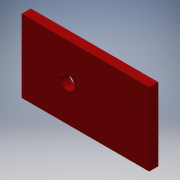
# Autodesk Inventor part: Gripper Piston
Saved by Autodesk Inventor 2016 (Build 200138000, 138)
## iProperties
Created: 2015-06-19
Part Number: Gripper Piston
Material: Aluminum 6061
Document SubType Name: Modeling
Designer: steele
Density: 2.7 g/cm^3
Appearance: Red
Mass: 71.2341 g
Surface Area: 102.839 cm^2
Volume: 26.383 cm^3
Author: steele
Autodesk Inventor part; units mm, degrees
ref_plane "YZ Plane" through (0, 0, 0) normal (1, 0, 0) x (0, 1, 0)
ref_plane "XZ Plane" through (0, 0, 0) normal (0, 1, 0) x (-1, 0, 0)
ref_plane "XY Plane" through (0, 0, 0) normal (0, 0, 1) x (1, 0, 0)
sketch "Sketch2" plane through (0, 0, 0) normal (0, 0, 1) x (1, 0, 0)
  line L0 (0, 0) -> (-31.75, 0) construction
  line L1 (-31.75, 0) -> (-31.75, -25.4)
  line L2 (-31.75, 0) -> (-31.75, 25.4)
  line L3 (-31.75, 25.4) -> (57.15, 25.4)
  line L4 (0, 0) -> (0, -25.4) construction
  line L5 (0, 0) -> (57.15, 0) construction
  line L6 (-31.75, -25.4) -> (57.15, -25.4)
  line L7 (57.15, 25.4) -> (57.15, -25.4)
  dimension "edgeToCenterOfPiston" = 31.75
  dimension "heiight" = 50.8
  dimension "width" = 88.9
  dimension "d7" = 88.9
  dimension "d8" = 88.9
  constraints: 16 end point, 4 horizontal, 3 vertical, 1 collinear, 1 parallel
  measures "edgeToCenterOfPiston" distance of L0.start L0.end
  measures "heiight" distance of L1.end L2.end
  measures "width" distance from line of L5.end L1
  measures "d7" distance of L2.end L3.end
  measures "d8" distance of L1.end L6.end
extrude "Extrusion1" add sketch "Sketch2" along normal mid plane 6.35
sketch "Sketch3" plane through (0, 0, 3.175) normal (0, 0, 1) x (1, 0, 0)
  circle A0 centre (0, 0) radius 5.0165
  dimension "d11" = 10.033
  constraints: 1 centre point, 1 coincident
  measures "d11" diameter of A0
extrude "Extrusion2" cut sketch "Sketch3" against normal through all
equation "\"d7\" = width"
equation "\"d8\" = width"
body "Solid1"
